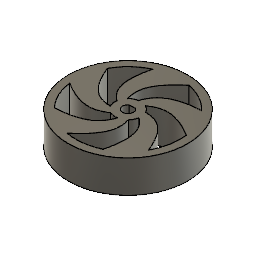
wheels_v1 (Autodesk Fusion 360 design; units mm, degrees)
Autodesk Fusion 360 part; units mm, degrees
note: some values were not read from the file. Set by a fixed rule: which sketch regions a step uses.
sketch "Sketch1" plane through (0, 0, 0) normal (0, 1, 0) x (1, 0, 0)
  circle A0 centre (0, 0) radius 2.5
  circle A1 centre (0, 0) radius 27.5
  circle A2 centre (0, 0) radius 6
  circle A3 centre (0, 0) radius 24
  line L0 (0, 0) -> (0, 2.5)
  line L1 (-1.5, 2) -> (1.5, 2)
  line L2 (1.5, 2) -> (1.5, -2)
  line L3 (1.5, -2) -> (-1.5, -2)
  line L4 (-1.5, -2) -> (-1.5, 2)
  line L5 (0, 0) -> (0, -2.5)
  spline S0 degree 5 poles (-10.2165, 21.7169) (-10.3629, 21.1355) (-10.6365, 19.9863) (-10.9889, 18.3035) (-11.3409, 16.1432) (-11.5701, 13.5918) (-11.567, 11.2048) (-11.3076, 8.9989) (-10.7716, 6.9887) (-9.9564, 5.1759) (-8.8773, 3.5497) (-7.8173, 2.3879) (-6.9183, 1.5901) (-6.2735, 1.0903) (-5.9397, 0.8485) knots 0 0 0 0 0 0 0.1 0.2 0.3 0.4 0.5 0.6 0.7 0.8 0.9 1 1 1 1 1 1
  spline S1 degree 5 poles (-21.0302, 11.5643) (-20.8069, 11.0078) (-20.3528, 9.9173) (-19.6488, 8.3487) (-18.6637, 6.3941) (-17.3495, 4.1953) (-15.9439, 2.2659) (-14.4375, 0.6338) (-12.8223, -0.6775) (-11.0972, -1.6649) (-9.2683, -2.3461) (-7.7279, -2.6631) (-6.5316, -2.7801) (-5.7162, -2.8054) (-5.3041, -2.8048) knots 0 0 0 0 0 0 0.1 0.2 0.3 0.4 0.5 0.6 0.7 0.8 0.9 1 1 1 1 1 1
  spline S2 degree 5 poles (-23.8111, -3.0055) (-23.3034, -3.3245) (-22.295, -3.9398) (-20.8034, -4.795) (-18.8576, -5.7973) (-16.502, -6.8037) (-14.2308, -7.5384) (-12.0527, -7.9734) (-9.9752, -8.0848) (-7.9993, -7.8697) (-6.1192, -7.3459) (-4.6867, -6.6968) (-3.6501, -6.0883) (-2.9756, -5.6295) (-2.6425, -5.3868) knots 0 0 0 0 0 0 0.1 0.2 0.3 0.4 0.5 0.6 0.7 0.8 0.9 1 1 1 1 1 1
  spline S3 degree 5 poles (-17.4969, -16.4273) (-16.8987, -16.3869) (-15.7212, -16.292) (-14.0119, -16.1072) (-11.8486, -15.7743) (-9.3513, -15.2039) (-7.082, -14.4633) (-5.0642, -13.535) (-3.318, -12.4041) (-1.8458, -11.0686) (-0.6328, -9.5397) (0.1447, -8.1726) (0.6256, -7.0711) (0.9016, -6.3034) (1.0285, -5.9112) knots 0 0 0 0 0 0 0.1 0.2 0.3 0.4 0.5 0.6 0.7 0.8 0.9 1 1 1 1 1 1
  spline S4 degree 5 poles (-4.4996, -23.5744) (-4.0393, -23.1901) (-3.1425, -22.4212) (-1.8683, -21.267) (-0.3138, -19.7261) (1.3713, -17.7968) (2.7719, -15.8637) (3.8587, -13.9267) (4.6066, -11.9854) (5.0126, -10.0396) (5.0954, -8.0897) (4.9208, -6.5267) (4.6624, -5.3529) (4.4345, -4.5696) (4.3066, -4.1777) knots 0 0 0 0 0 0 0.1 0.2 0.3 0.4 0.5 0.6 0.7 0.8 0.9 1 1 1 1 1 1
  spline S5 degree 5 poles (10.2165, -21.7169) (10.3629, -21.1355) (10.6365, -19.9863) (10.9889, -18.3035) (11.3409, -16.1432) (11.5701, -13.5918) (11.567, -11.2048) (11.3076, -8.9989) (10.7716, -6.9887) (9.9564, -5.1759) (8.8773, -3.5497) (7.8173, -2.3879) (6.9183, -1.5901) (6.2735, -1.0903) (5.9397, -0.8485) knots 0 0 0 0 0 0 0.1 0.2 0.3 0.4 0.5 0.6 0.7 0.8 0.9 1 1 1 1 1 1
  spline S6 degree 5 poles (21.0302, -11.5643) (20.8069, -11.0078) (20.3528, -9.9173) (19.6488, -8.3487) (18.6637, -6.3941) (17.3495, -4.1953) (15.9439, -2.2659) (14.4375, -0.6338) (12.8223, 0.6775) (11.0972, 1.6649) (9.2683, 2.3461) (7.7279, 2.6631) (6.5316, 2.7801) (5.7162, 2.8054) (5.3041, 2.8048) knots 0 0 0 0 0 0 0.1 0.2 0.3 0.4 0.5 0.6 0.7 0.8 0.9 1 1 1 1 1 1
  spline S7 degree 5 poles (23.8111, 3.0055) (23.3034, 3.3245) (22.295, 3.9398) (20.8034, 4.795) (18.8576, 5.7973) (16.502, 6.8037) (14.2308, 7.5384) (12.0527, 7.9734) (9.9752, 8.0848) (7.9993, 7.8697) (6.1192, 7.3459) (4.6867, 6.6968) (3.6501, 6.0883) (2.9756, 5.6295) (2.6425, 5.3868) knots 0 0 0 0 0 0 0.1 0.2 0.3 0.4 0.5 0.6 0.7 0.8 0.9 1 1 1 1 1 1
  spline S8 degree 5 poles (17.4969, 16.4273) (16.8987, 16.3869) (15.7212, 16.292) (14.0119, 16.1072) (11.8486, 15.7743) (9.3513, 15.2039) (7.082, 14.4633) (5.0642, 13.535) (3.318, 12.4041) (1.8458, 11.0686) (0.6328, 9.5397) (-0.1447, 8.1726) (-0.6256, 7.0711) (-0.9016, 6.3034) (-1.0285, 5.9112) knots 0 0 0 0 0 0 0.1 0.2 0.3 0.4 0.5 0.6 0.7 0.8 0.9 1 1 1 1 1 1
  spline S9 degree 5 poles (4.4996, 23.5744) (4.0393, 23.1901) (3.1425, 22.4212) (1.8683, 21.267) (0.3138, 19.7261) (-1.3713, 17.7968) (-2.7719, 15.8637) (-3.8587, 13.9267) (-4.6066, 11.9854) (-5.0126, 10.0396) (-5.0954, 8.0897) (-4.9208, 6.5267) (-4.6624, 5.3529) (-4.4345, 4.5696) (-4.3066, 4.1777) knots 0 0 0 0 0 0 0.1 0.2 0.3 0.4 0.5 0.6 0.7 0.8 0.9 1 1 1 1 1 1
  dimension "d1" = 5
  dimension "d2" = 55
  dimension "d3" = 12
  dimension "d4" = 48
  dimension "d5" = 0.5
  dimension "d6" = 0.5
  dimension "d8" = 360
  measures "d1" diameter of A0
  measures "d2" diameter of A1
  measures "d3" diameter of A2
  measures "d4" diameter of A3
  measures "d5" distance of L1
  measures "d6" distance of L3
extrude "Extrude1" add sketch "Sketch1" along normal blind 15 contours A0 L0 L1 | A0 L0 L1 | A1 | A2 | A2 A3 S5 S6 | A2 A3 S7 S8 | A2 A3 S3 S4 | A2 A3 S0 S9 | A2 A3 S1 S2
